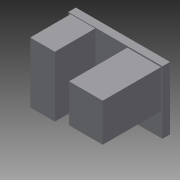
# Autodesk Inventor part: ccpad
Saved by Autodesk Inventor 2013 SP2 (Build 170200200, 200)
## iProperties
Created: 2019-01-29
Part Number: ccpad
Material: Generic
Document SubType Name: Modeling
Designer: alex
Density: 1 g/cm^3
Author: alex
Autodesk Inventor part; units mm, degrees
ref_plane "YZ Plane" through (0, 0, 0) normal (1, 0, 0) x (0, 1, 0)
ref_plane "XZ Plane" through (0, 0, 0) normal (0, 1, 0) x (-1, 0, 0)
ref_plane "XY Plane" through (0, 0, 0) normal (0, 0, 1) x (1, 0, 0)
sketch "Sketch1" plane through (0, 0, 0) normal (0, 1, 0) x (-1, 0, 0)
  line L0 (0, 0) -> (-21, 0)
  line L1 (-21, 0) -> (-21, -14)
  line L2 (-21, -14) -> (0, -14)
  line L3 (0, -14) -> (0, 0)
  dimension "d0" = 21
  dimension "d1" = 14
  constraints: 8 end point, 2 parallel, 1 horizontal, 1 perpendicular
  measures "d0" distance of L2.end L1.end
  measures "d1" distance of L1.end L0.end
extrude "Extrusion1" add sketch "Sketch1" along normal blind 1.7
sketch "Sketch2" plane through (0, 0, 0) normal (0, -1, 0) x (1, 0, 0)
  line L0 (0, 0) -> (21, 0) projected
  line L1 (0, -14) -> (0, 0) projected
  line L2 (-4.6, 0) -> (27.6, 0) projected
  line L3 (0, -16.8) -> (0, 2.8) projected
  line L4 (0.52, -0.17) -> (6.02, -0.17)
  line L5 (6.02, -0.17) -> (6.02, -13.67)
  line L6 (6.02, -13.67) -> (0.52, -13.67)
  line L7 (0.52, -13.67) -> (0.52, -0.17)
  line L8 (2, -1.84) -> (2, -0.17)
  line L9 (2, -1.84) -> (0.52, -1.84)
  line L10 (4.54, -12) -> (4.54, -13.67)
  line L11 (4.54, -12) -> (6.02, -12)
  point P0 (4.54, -1.84)
  point P1 (2, -4.38)
  point P2 (4.54, -4.38)
  point P3 (2, -6.92)
  point P4 (4.54, -6.92)
  point P5 (2, -9.46)
  point P6 (4.54, -9.46)
  point P7 (2, -12)
  dimension "d12" = 2.54
  dimension "d15" = 2.54
  dimension "d18" = 5.5
  dimension "d19" = 13.5
  dimension "d20" = 4.38
  dimension "d21" = 4.54
  constraints: 16 end point, 5 perpendicular, 4 parallel, 4 point on line, 2 horizontal, 1 vertical, 9 other
  measures "d12" distance of L8.start point (4.54, -1.84)
  measures "d15" distance of L8.start point (2, -4.38)
  measures "d18" distance of L5.end L6.end
  measures "d19" distance of L4.end L5.end
  measures "d20" distance from line of L0 point (4.54, -4.38)
  measures "d21" distance from line of L1 point (4.54, -4.38)
extrude "Extrusion2" add sketch "Sketch2" along normal blind 9
sketch "Sketch3" plane through (0, 0, 0) normal (0, -1, 0) x (1, 0, 0)
  line L0 (0, -14) -> (0, 0) projected
  line L1 (13.1877, -8.8011) -> (20.6877, -8.8011)
  line L2 (20.6877, -8.8011) -> (20.6877, -0.3011)
  line L3 (20.6877, -0.3011) -> (13.1877, -0.3011)
  line L4 (13.1877, -0.3011) -> (13.1877, -8.8011)
  line L5 (19.1, -2.8011) -> (19.1, -0.3011)
  line L6 (19.1, -6.3011) -> (19.1, -8.8011)
  dimension "d25" = 19.1
  dimension "d26" = 3.5
  dimension "d27" = 7.5
  dimension "d28" = 8.5
  constraints: 12 end point, 3 perpendicular, 2 parallel, 2 point on line, 1 collinear, 1 horizontal, 1 vertical alignment
  measures "d25" distance from line of L0 L5.start
  measures "d26" distance of L5.start L6.start
  measures "d27" distance of L2.end L3.end
  measures "d28" distance of L3.end L1.start
extrude "Extrusion3" add sketch "Sketch3" along normal blind 13
body "Solid1"
